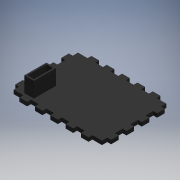
# Autodesk Inventor part: bottom
Saved by Autodesk Inventor 2019 (Build 230136000, 136)
## iProperties
Created: 2018-06-07
Part Number: bottom
Material: PBT Plastic Black
Document SubType Name: Modeling
Designer: stra92745
Density: 1.31 g/cm^3
Appearance: Smooth - White
Author: stra92745
Autodesk Inventor part; units mm, degrees
ref_plane "YZ Plane" through (0, 0, 0) normal (1, 0, 0) x (0, 1, 0)
ref_plane "XZ Plane" through (0, 0, 0) normal (0, 1, 0) x (-1, 0, 0)
ref_plane "XY Plane" through (0, 0, 0) normal (0, 0, 1) x (1, 0, 0)
sketch "Sketch1" plane through (0, 0, 0) normal (0, 1, 0) x (-1, 0, 0)
  line L0 (0, 0) -> (-100, 0)
  line L1 (-100, 0) -> (-100, -75)
  line L2 (-100, -75) -> (0, -75)
  line L3 (0, -75) -> (0, 0)
  dimension "d0" = 100
  dimension "d1" = 75
  constraints: 8 end point, 2 parallel, 1 horizontal, 1 perpendicular
  measures "d0" distance of L2.end L1.end
  measures "d1" distance of L1.end L0.end
extrude "Extrusion1" add sketch "Sketch1" along normal blind 4
sketch "Sketch3" plane through (0, 4, 0) normal (0, 1, 0) x (1, 0, 0)
  line L0 (100, 75) -> (0, 75) construction
  line L1 (0, 75) -> (0, 0) construction
  line L2 (0, 0) -> (100, 0) construction
  line L3 (100, 0) -> (100, 75) construction
  line L4 (4, 71) -> (96, 71) construction
  line L5 (96, 71) -> (96, 4) construction
  line L6 (96, 4) -> (4, 4) construction
  line L7 (4, 4) -> (4, 71) construction
  line L8 (0, 37.5) -> (100, 37.5) construction
  line L9 (50, 75) -> (50, 0) construction
  line L10 (0, 65.5) -> (4, 65.5)
  line L11 (4, 65.5) -> (4, 71)
  line L12 (4, 71) -> (14, 71)
  line L13 (14, 71) -> (14, 75)
  line L14 (14, 75) -> (0, 75)
  line L15 (0, 75) -> (0, 65.5)
  line L16 (0, 57.5) -> (4, 57.5)
  line L17 (4, 57.5) -> (4, 49.5)
  line L18 (4, 49.5) -> (0, 49.5)
  line L19 (0, 49.5) -> (0, 57.5)
  line L20 (0, 41.5) -> (4, 41.5)
  line L21 (4, 37.5) -> (4, 41.5)
  line L22 (0, 41.5) -> (0, 37.5)
  line L23 (22, 75) -> (22, 71)
  line L24 (22, 71) -> (30, 71)
  line L25 (30, 71) -> (30, 75)
  line L26 (30, 75) -> (22, 75)
  line L27 (38, 75) -> (38, 71)
  line L28 (38, 71) -> (46, 71)
  line L29 (46, 71) -> (46, 75)
  line L30 (46, 75) -> (38, 75)
  line L31 (0, 9.5) -> (4, 9.5)
  line L32 (4, 9.5) -> (4, 4)
  line L33 (4, 4) -> (14, 4)
  line L34 (14, 4) -> (14, 0)
  line L35 (14, 0) -> (0, 0)
  line L36 (0, 0) -> (0, 9.5)
  line L37 (0, 17.5) -> (4, 17.5)
  line L38 (4, 17.5) -> (4, 25.5)
  line L39 (4, 25.5) -> (0, 25.5)
  line L40 (0, 25.5) -> (0, 17.5)
  line L41 (0, 33.5) -> (4, 33.5)
  line L42 (4, 37.5) -> (4, 33.5)
  line L43 (0, 33.5) -> (0, 37.5)
  line L44 (22, 0) -> (22, 4)
  line L45 (22, 4) -> (30, 4)
  line L46 (30, 4) -> (30, 0)
  line L47 (30, 0) -> (22, 0)
  line L48 (38, 0) -> (38, 4)
  line L49 (38, 4) -> (46, 4)
  line L50 (46, 4) -> (46, 0)
  line L51 (46, 0) -> (38, 0)
  line L52 (100, 75) -> (100, 0) construction
  line L53 (96, 4) -> (96, 71) construction
  line L54 (100, 65.5) -> (96, 65.5)
  line L55 (96, 65.5) -> (96, 71)
  line L56 (96, 71) -> (86, 71)
  line L57 (86, 71) -> (86, 75)
  line L58 (86, 75) -> (100, 75)
  line L59 (100, 75) -> (100, 65.5)
  line L60 (100, 57.5) -> (96, 57.5)
  line L61 (96, 57.5) -> (96, 49.5)
  line L62 (96, 71) -> (96, 4)
  line L63 (96, 49.5) -> (100, 49.5)
  line L64 (100, 49.5) -> (100, 57.5)
  line L65 (100, 41.5) -> (96, 41.5)
  line L66 (96, 37.5) -> (96, 41.5)
  line L67 (100, 41.5) -> (100, 37.5)
  line L68 (78, 75) -> (78, 71)
  line L69 (78, 71) -> (70, 71)
  line L70 (70, 71) -> (70, 75)
  line L71 (70, 75) -> (78, 75)
  line L72 (62, 75) -> (62, 71)
  line L73 (62, 71) -> (54, 71)
  line L74 (54, 71) -> (54, 75)
  line L75 (54, 75) -> (62, 75)
  line L76 (78, 0) -> (78, 4)
  line L77 (70, 4) -> (70, 0)
  line L78 (78, 4) -> (70, 4)
  line L79 (70, 0) -> (78, 0)
  line L80 (54, 4) -> (54, 0)
  line L81 (62, 4) -> (54, 4)
  line L82 (54, 0) -> (62, 0)
  line L83 (62, 0) -> (62, 4)
  line L84 (96, 4) -> (86, 4)
  line L85 (100, 9.5) -> (96, 9.5)
  line L86 (96, 9.5) -> (96, 4)
  line L87 (86, 4) -> (86, 0)
  line L88 (86, 0) -> (100, 0)
  line L89 (96, 17.5) -> (96, 25.5)
  line L90 (100, 17.5) -> (96, 17.5)
  line L91 (96, 25.5) -> (100, 25.5)
  line L92 (96, 37.5) -> (96, 33.5)
  line L93 (100, 33.5) -> (96, 33.5)
  line L94 (100, 33.5) -> (100, 37.5)
  line L95 (100, 25.5) -> (100, 17.5)
  line L96 (100, 0) -> (100, 9.5)
  dimension "d9" = 8
  dimension "d11" = 4
  dimension "d12" = 8
  dimension "d13" = 8
  dimension "d14" = 8
  dimension "d15" = 8
  dimension "d16" = 8
  dimension "d17" = 4
  dimension "d18" = 8
  dimension "d22" = 4
  constraints: 186 end point, 55 symmetric about line, 19 point on line, 9 collinear, 7 perpendicular, 4 midpoint, 1 parallel, 1 vertical, 3 other
  measures "d9" distance between parallel lines of L16 L10
  measures "d11" distance between parallel lines of L8 L20
  measures "d12" distance between parallel lines of L20 L18
  measures "d13" distance between parallel lines of L16 L18
  measures "d14" distance of L25.end L23.start
  measures "d15" distance between parallel lines of L25 L27
  measures "d16" distance of L29.end L27.start
  measures "d17" distance between parallel lines of L9 L29
  measures "d18" distance between parallel lines of L13 L23
  measures "d22" distance between parallel lines of L0 L4
extrude "Extrusion3" cut sketch "Sketch3" against normal up to surface (4 mm away)
sketch "Sketch4" plane through (0, 4, 0) normal (0, 1, 0) x (1, 0, 0)
  line L0 (14, 28) -> (21, 28)
  line L1 (21, 28) -> (21, 8)
  line L2 (21, 8) -> (14, 8)
  line L3 (14, 8) -> (14, 28)
  line L4 (78, 0) -> (86, 0) projected
  line L5 (0, 33.5) -> (0, 25.5) projected
  point P0 (0, 0)
  dimension "d23" = 7
  dimension "d24" = 20
  dimension "d26" = 8
  dimension "d32" = 14
  constraints: 8 end point, 2 parallel, 1 horizontal, 1 perpendicular
  measures "d23" distance of L1.end L2.end
  measures "d24" distance of L0.end L1.end
  measures "d26" distance between parallel lines of L4 L2
  measures "d32" distance between parallel lines of L5 L3
extrude "Extrusion4" cut sketch "Sketch4" against normal up to surface (4 mm away)
sketch "Sketch5" plane through (0, 4, 0) normal (0, 1, 0) x (1, 0, 0)
  line L0 (14, 8) -> (14, 28) projected
  line L1 (14, 28) -> (21, 28) projected
  line L2 (21, 28) -> (21, 8) projected
  line L3 (21, 8) -> (14, 8) projected
  line L4 (22.5, 29.5) -> (12.5, 29.5)
  line L5 (12.5, 29.5) -> (12.5, 6.5)
  line L6 (12.5, 6.5) -> (22.5, 6.5)
  line L7 (22.5, 6.5) -> (22.5, 29.5)
  point P0 (0, 0)
  dimension "d29" = 1.5
  constraints: 8 end point, 3 other
  measures "d29" distance between parallel lines of L1 L4
extrude "Extrusion5" add sketch "Sketch5" along normal blind 16
body "Solid1"
